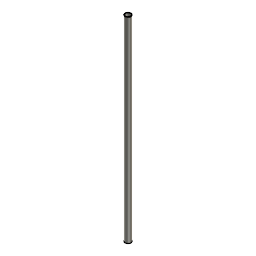
Assem1 final prj (Autodesk Fusion 360 archive; units mm, degrees)
design "Carbon Fiber Tube 52.7cm height 15mm OD 2mm thickness"
Autodesk Fusion 360 part; units mm, degrees
sketch "Sketch1" plane through (0, 0, 0) normal (0, 0, 1) x (1, 0, 0)
  circle A0 centre (0, 0) radius 7.5
  circle A1 centre (0, 0) radius 6.5
  dimension "d1" = 15
  dimension "d2" = -1
  constraint coincident A0.centre A1.centre
  measures "d1" diameter of A0
extrude "Extrude1" add sketch "Sketch1" along normal blind 497
equation "d3 = 527 mm - 30 mm"

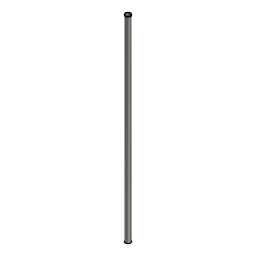
design "Carbon Fiber Tube 56cm length 15mm OD 1mm thickness"
Autodesk Fusion 360 part; units mm, degrees
sketch "Sketch1" plane through (0, 0, 0) normal (0, 0, 1) x (1, 0, 0)
  circle A0 centre (0, 0) radius 7.5
  circle A1 centre (0, 0) radius 6.5
  dimension "d1" = 15
  dimension "d2" = -1
  constraint coincident A0.centre A1.centre
  measures "d1" diameter of A0
extrude "Extrude1" add sketch "Sketch1" along normal blind 530
equation "d3 = 560 mm - 30 mm"

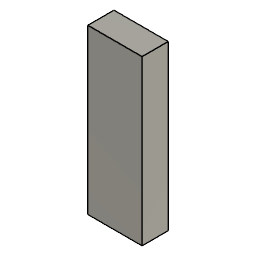
design "Lipo 10K mah cad"
Autodesk Fusion 360 part; units mm, degrees
sketch "Sketch1" plane through (0, 0, 0) normal (0, 0, 1) x (1, 0, 0)
  line L0 (-29, 14) -> (29, 14)
  line L1 (29, 14) -> (29, -14)
  line L2 (29, -14) -> (-29, -14)
  line L3 (-29, -14) -> (-29, 14)
  line L4 (-29, 14) -> (29, -14) construction
  line L5 (29, 14) -> (-29, -14) construction
  dimension "d1" = 28
  dimension "d2" = 58
  constraint horizontal L0
  constraint perpendicular L0 L1
  constraint parallel L0 L2
  constraint parallel L1 L3
  constraint coincident L4 origin
  constraint coincident L5 origin
  measures "d1" distance of L0.start L2.end
  measures "d2" distance of L0.start L0.end
extrude "Extrude1" add sketch "Sketch1" along normal blind 175

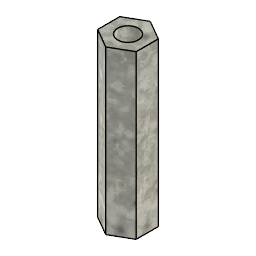
design "Layer 0 Bottom spacer"
Autodesk Fusion 360 part; units mm, degrees
sketch "Sketch1" plane through (0, 0, 0) normal (0, 0, 1) x (1, 0, 0)
  circle A0 centre (0, 0) radius 1.6
  line L0 (-3, -1.7321) -> (0, -3.4641)
  line L1 (0, -3.4641) -> (3, -1.7321)
  line L2 (3, -1.7321) -> (3, 1.7321)
  line L3 (3, 1.7321) -> (0, 3.4641)
  line L4 (0, 3.4641) -> (-3, 1.7321)
  line L5 (-3, 1.7321) -> (-3, -1.7321)
  dimension "d1" = 3.2
  constraint coincident A0.centre origin
  measures "d1" diameter of A0
extrude "Extrude1" add sketch "Sketch1" along normal blind 25.3
